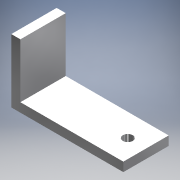
# Autodesk Inventor part: Small connector
Saved by Autodesk Inventor 2019.4 (Build 234330000, 330)
## iProperties
Created: 2020-01-31
Part Number: Small connector
Material: Aluminum 6061
Document SubType Name: Modeling
Designer: Mark
Mass: 27.5818 g
Surface Area: 51.5344 cm^2
Volume: 10.2155 cm^3
Density: 2.7 g/cm^3
Appearance: Aluminum - Flat
Author: Mark
Autodesk Inventor part; units mm, degrees
ref_plane "YZ Plane" through (0, 0, 0) normal (1, 0, 0) x (0, 1, 0)
ref_plane "XZ Plane" through (0, 0, 0) normal (0, 1, 0) x (-1, 0, 0)
ref_plane "XY Plane" through (0, 0, 0) normal (0, 0, 1) x (1, 0, 0)
sketch "Sketch1" plane through (0, 0, 0) normal (0, 0, 1) x (1, 0, 0)
  line L0 (0, 0) -> (61.724, 0)
  line L1 (61.724, 0) -> (61.724, 4)
  line L2 (61.724, 4) -> (0, 4)
  line L3 (0, 4) -> (0, 0)
  line L4 (0, 4) -> (4, 4)
  line L5 (4, 4) -> (4, 34)
  line L6 (4, 34) -> (0, 34)
  line L7 (0, 34) -> (0, 4)
  dimension "d0" = 61.724
  dimension "d1" = 4
  dimension "d2" = 4
  dimension "d3" = 30
  constraints: 16 end point, 4 parallel, 2 horizontal, 2 perpendicular
  measures "d0" distance of L2.end L1.end
  measures "d1" distance of L1.end L0.end
  measures "d2" distance of L6.end L5.end
  measures "d3" distance of L5.end L4.end
extrude "Extrusion1" add sketch "Sketch1" along normal blind 25
sketch "Sketch2" plane through (4, 4, 0) normal (0, 1, 0) x (1, 0, 0)
  circle A0 centre (47.724, -12.5) radius 2.75
  line L0 (57.724, 0) -> (57.724, -25) projected
  line L1 (57.724, 0) -> (0, 0) projected
  point P0 (-4, 0)
  dimension "d6" = 5.5
  dimension "d7" = 10
  dimension "d8" = 12.5
  constraints: 1 centre point
  measures "d6" diameter of A0
  measures "d7" distance from line of L0 A0.centre
  measures "d8" distance from line of L1 A0.centre
extrude "Extrusion2" cut sketch "Sketch2" against normal blind 25
sketch "Sketch3" plane through (0, 0, 0) normal (-1, 0, 0) x (0, 0, 1)
  circle A0 centre (12.5, 10) radius 2.75
  circle A1 centre (12.5, 25) radius 2.75
  line L0 (0, 0) -> (25, 0) projected
  line L1 (0, 0) -> (0, 34) projected
  dimension "d11" = 5.5
  dimension "d12" = 5.5
  dimension "d13" = 10
  dimension "d14" = 15
  dimension "d15" = 12.5
  dimension "d16" = 12.5
  constraints: 2 centre point
  measures "d11" diameter of A0
  measures "d12" diameter of A1
  measures "d13" distance from line of L0 A0.centre
  measures "d14" distance of A1.centre A0.centre
  measures "d15" distance from line of L1 A0.centre
  measures "d16" distance from line of L1 A1.centre
extrude "Extrusion3" cut sketch "Sketch3" against normal blind 25
body "Solid1"
